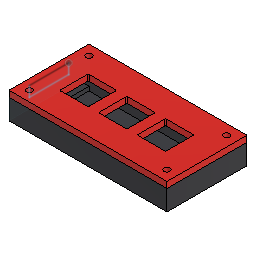
macropad v1.2 (Autodesk Fusion 360 design; units mm, degrees)
part number: 2026-06-06-15-26-31-793
Autodesk Fusion 360 part; units mm, degrees
sketch "base" plane through (0, 0, 0) normal (0, 0, 1) x (1, 0, 0)
  circle A0 centre (-5, -5) radius 1.45
  circle A1 centre (62.8, -5) radius 1.45
  line L0 (28.9, 29.4) -> (28.9, -10) construction
  line L1 (0, 0) -> (57.8, 0)
  circle A2 centre (-5, 24.4) radius 1.45
  circle A3 centre (62.8, 24.4) radius 1.45
  line L2 (67.8, 29.4) -> (67.8, -10)
  line L3 (57.8, 0) -> (57.8, 19.4)
  line L4 (67.8, -10) -> (-10, -10)
  line L5 (57.8, 19.4) -> (0, 19.4)
  line L6 (-10, 29.4) -> (67.8, 29.4)
  line L7 (-10, -10) -> (-10, 29.4)
  line L8 (0, 19.4) -> (0, 0)
  line L9 (67.8, 9.7) -> (-10, 9.7) construction
  dimension "d12" = 19.4
  dimension "d13" = 57.8
  dimension "d14" = 10
  dimension "d15" = 10
  dimension "d16" = 10
  dimension "d17" = 10
  dimension "d18" = 2.9
  dimension "d19" = 5
  dimension "d20" = 5
  constraint horizontal L1
  constraint vertical L3
  constraint horizontal L5
  constraint vertical L8
  constraint coincident L1.start L8.end
  constraint horizontal L6
  constraint vertical L2
  constraint horizontal L4
  constraint vertical L7
  constraint midpoint L0.start L6
  constraint midpoint L0.end L4
  constraint midpoint L9.start L2
  constraint midpoint L9.end L7
  constraint symmetric L0 A2 A3
  constraint symmetric A0 A2 L9
  constraint symmetric A1 A3 L9
  measures "d12" distance of L1.start L5.end
  measures "d13" distance of L1.start L1.end
  measures "d14" distance of L5 L6
  measures "d15" distance of L2 L3
  measures "d16" distance of L1 L4
  measures "d17" distance of L7 L8
  measures "d18" diameter of A2
  measures "d19" distance of A2.centre L6
  measures "d20" distance of A2.centre L7
extrude "Extrude2" add sketch "base" along normal blind 3 contours L1 L3 L5 L8 | L2 L4 L6 L7 makes body 1
extrude "Extrude3" add sketch "base" along normal blind 10 bodies 1
sketch "plate-2026-06-06T10_45_52.684Z" plane through (0, 0, 10) normal (0, 0, 1) x (1, 0, 0)
  line L0 (3.025, 16.475) -> (16.025, 16.475)
  line L1 (3.025, 2.475) -> (16.025, 2.475)
  line L2 (2.525, 15.975) -> (2.525, 2.975)
  line L3 (16.525, 15.975) -> (16.525, 2.975)
  arc A0 (3.025, 16.475) -> (2.525, 15.975) centre (3.025, 15.975) ccw
  arc A1 (16.525, 15.975) -> (16.025, 16.475) centre (16.025, 15.975) ccw
  arc A2 (2.525, 2.975) -> (3.025, 2.475) centre (3.025, 2.975) ccw
  arc A3 (16.025, 2.475) -> (16.525, 2.975) centre (16.025, 2.975) ccw
  line L4 (22.075, 16.475) -> (35.075, 16.475)
  line L5 (22.075, 2.475) -> (35.075, 2.475)
  line L6 (21.575, 15.975) -> (21.575, 2.975)
  line L7 (35.575, 15.975) -> (35.575, 2.975)
  arc A4 (22.075, 16.475) -> (21.575, 15.975) centre (22.075, 15.975) ccw
  arc A5 (35.575, 15.975) -> (35.075, 16.475) centre (35.075, 15.975) ccw
  arc A6 (21.575, 2.975) -> (22.075, 2.475) centre (22.075, 2.975) ccw
  arc A7 (35.075, 2.475) -> (35.575, 2.975) centre (35.075, 2.975) ccw
  line L8 (41.125, 16.475) -> (54.125, 16.475)
  line L9 (41.125, 2.475) -> (54.125, 2.475)
  line L10 (40.625, 15.975) -> (40.625, 2.975)
  line L11 (54.625, 15.975) -> (54.625, 2.975)
  arc A8 (41.125, 16.475) -> (40.625, 15.975) centre (41.125, 15.975) ccw
  arc A9 (54.625, 15.975) -> (54.125, 16.475) centre (54.125, 15.975) ccw
  arc A10 (40.625, 2.975) -> (41.125, 2.475) centre (41.125, 2.975) ccw
  arc A11 (54.125, 2.475) -> (54.625, 2.975) centre (54.125, 2.975) ccw
  line L12 (0, -0.05) -> (59.2084, -0.05)
  line L13 (0, 22.8962) -> (59.2084, 22.8962)
  line L14 (0, -0.05) -> (0, 22.8962)
  line L15 (59.2084, -0.05) -> (59.2084, 22.8962)
extrude "Extrude4" add sketch "plate-2026-06-06T10_45_52.684Z" 1 faces at (19.2667, -3.7528, 10) along normal blind 3 separate body on bodies 1 makes body 2
sketch "Sketch5" plane through (-10, 0, 0) normal (-1, 0, 0) x (0, -1, 0)
  line L0 (-29.4, 0) -> (10, 0)
  line L1 (10, 0) -> (10, 10)
  line L2 (10, 10) -> (-29.4, 10)
  line L3 (-29.4, 10) -> (-29.4, 0)
  line L4 (0, 5) -> (-19.4, 5)
  line L5 (-19.4, 5) -> (-19.4, 10)
  line L6 (-19.4, 10) -> (0, 10)
  line L7 (0, 10) -> (0, 5)
  dimension "d29" = 19.4
  constraint horizontal L4
  constraint vertical L5
  constraint horizontal L6
  constraint vertical L7
  constraint coincident L2 L5.end
  measures "d29" distance of L4.start L4.end
extrude "Extrude6" cut sketch "Sketch5" against normal blind 12 contours L2 L4 L5 L6 L7 bodies 1
named bodies: "base", "cover"
